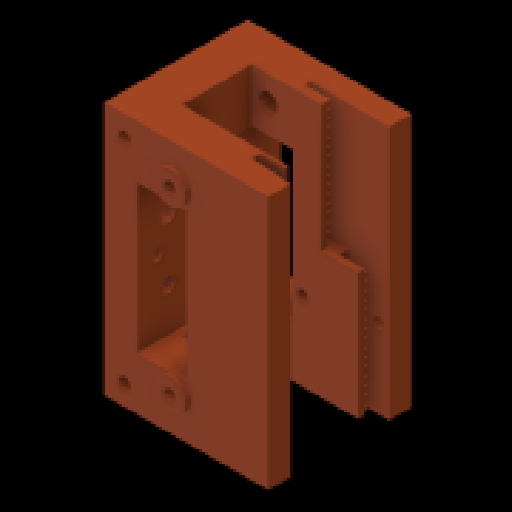
# Autodesk Inventor part: Toolhead Base
Saved by Autodesk Inventor 2023.3 (Build 273359000, 359)
## iProperties
Created: 2023-02-04
Part Number: Toolhead Base
Material: ABS Plastic
Document SubType Name: Modeling
Designer: remop
Density: 1.06 g/cm^3
Appearance: Smooth - Light Orange
Author: remop
Autodesk Inventor part; units mm, degrees
ref_plane "YZ Plane" through (0, 0, 0) normal (1, 0, 0) x (0, 1, 0)
ref_plane "XZ Plane" through (0, 0, 0) normal (0, 1, 0) x (-1, 0, 0)
ref_plane "XY Plane" through (0, 0, 0) normal (0, 0, 1) x (1, 0, 0)
sketch "Sketch1" plane through (0, 0, 0) normal (0, 0, 1) x (1, 0, 0)
  circle A0 centre (42.2396, 26.5) radius 2.25 projected
  circle A1 centre (42.2396, -23.5) radius 2.25 projected
  circle A2 centre (42.2396, -23.5) radius 6
  circle A3 centre (42.2396, 26.5) radius 6
  line L0 (48.2396, -23.5) -> (48.2396, -16.5)
  line L1 (48.2396, -16.5) -> (34.2396, -16.5)
  line L2 (34.2396, -16.5) -> (28.2396, -22.5)
  line L3 (28.2396, -22.5) -> (28.2396, -29.5)
  line L4 (28.2396, -29.5) -> (42.2396, -29.5)
  line L5 (48.2396, 26.5) -> (48.2396, 19.5)
  line L6 (48.2396, 19.5) -> (28.2396, 19.5)
  line L7 (28.2396, 19.5) -> (28.2396, 32.5)
  line L8 (28.2396, 32.5) -> (42.2396, 32.5)
  line L9 (42.2396, -29.5) -> (48.2396, -29.5)
  line L10 (48.2396, -29.5) -> (48.2396, -23.5)
  line L11 (48.2396, 26.5) -> (48.2396, 32.5)
  line L12 (48.2396, 32.5) -> (42.2396, 32.5)
  point P0 (0, 0)
  dimension "d0" = 12
  dimension "d3" = 14
  dimension "d4" = 45
  dimension "d5" = 7
  dimension "d6" = 7
  constraints: 26 end point, 8 tangent, 5 perpendicular, 5 point on circle, 3 horizontal, 2 centre point, 2 coincident, 2 point on line, 2 vertical, 1 collinear, 1 equal radius, 1 parallel, 1 vertical alignment
  measures "d0" diameter of A2
  measures "d3" distance of L3.end L4.end
  measures "d4" angle of L2 L3
  measures "d5" distance of L0.start L0.end
  measures "d6" distance of L2.end L3.end
extrude "Extrusion1" add sketch "Sketch1" along normal blind 9
sketch "Sketch2" plane through (0, 0, 9) normal (0, 0, 1) x (1, 0, 0)
  line L0 (28.2396, 32.5) -> (28.2396, 19.5) projected
  line L1 (28.2396, 19.5) -> (48.2396, 19.5) projected
  line L2 (48.2396, 19.5) -> (48.2396, 32.5) projected
  circle A0 centre (42.2396, 26.5) radius 2.25 projected
  line L3 (48.2396, -16.5) -> (34.2396, -16.5) projected
  line L4 (34.2396, -16.5) -> (28.2396, -22.5) projected
  line L5 (28.2396, -22.5) -> (28.2396, -29.5) projected
  line L6 (28.2396, -29.5) -> (48.2396, -29.5) projected
  circle A1 centre (42.2396, -23.5) radius 2.25 projected
  line L7 (36.2396, -15.705) -> (36.2396, 18.995) projected
  line L8 (36.2396, -15.705) -> (46.2396, -15.705) projected
  line L9 (46.2396, 18.995) -> (46.2396, -15.705) projected
  line L10 (36.2396, 18.995) -> (46.2396, 18.995) projected
  line L11 (34.2396, -16.5) -> (28.2396, -22.5) projected
  line L12 (28.2396, 19.5) -> (28.2396, -22.5)
  line L13 (36.2396, -15.705) -> (36.2396, -16.5)
  line L14 (36.2396, 18.995) -> (36.2396, 19.5)
  line L15 (28.2396, 19.5) -> (48.2396, 19.5) projected
  line L16 (38.2396, 19.5) -> (38.2396, 32.5)
  line L17 (48.2396, -16.5) -> (34.2396, -16.5) projected
  line L18 (38.2396, -16.5) -> (38.2396, -29.5)
  line L19 (28.2396, -29.5) -> (42.2396, -29.5) projected
  circle A2 centre (20.2396, -6.5) radius 14 projected
  circle A3 centre (20.2396, -6.5) radius 15
  line L20 (48.2396, -29.5) -> (48.2396, -16.5) projected
  line L21 (48.2396, 32.5) -> (28.2396, 32.5) projected
  point P0 (0, 0)
  point P1 (38.2396, 19.5)
  point P2 (35.2396, -6.5)
  point P3 (28.2396, -19.1886)
  point P4 (28.2396, 6.1886)
  dimension "d7" = 1
  constraints: 10 end point, 6 point on line, 2 midpoint, 1 centre point, 1 coincident, 1 collinear, 1 perpendicular, 1 vertical, 1 vertical alignment
  measures "d7" radial gap between concentric circles of A2 A3
extrude "Extrusion2" add sketch "Sketch2" along normal blind 10 contours L21 L16 L1 L0 | L1 L14 L7 L13 L3 L4 L12 A3 | L4 L3 L18 L6 L5
sketch "Sketch3" plane through (0, 0, 19) normal (0, 0, 1) x (1, 0, 0)
  line L0 (28.2396, -29.5) -> (38.2396, -29.5) projected
  line L1 (38.2396, -29.5) -> (38.2396, -16.5) projected
  line L2 (38.2396, -16.5) -> (36.2396, -16.5) projected
  line L3 (36.2396, -16.5) -> (36.2396, 19.5) projected
  line L4 (36.2396, 19.5) -> (38.2396, 19.5) projected
  line L5 (28.2396, 32.5) -> (28.2396, 6.1886) projected
  arc A0 (28.2396, -19.1886) -> (28.2396, 6.1886) centre (20.2396, -6.5) ccw projected
  line L6 (28.2396, -19.1886) -> (28.2396, -29.5) projected
  line L7 (28.2396, 19.5) -> (28.2396, 6.1886) projected
  line L8 (28.2396, -19.1886) -> (28.2396, -22.5) projected
  line L9 (28.2396, 6.1886) -> (28.2396, -19.1886)
  line L10 (38.2396, 32.5) -> (28.2396, 32.5) projected
  line L11 (38.2396, 19.5) -> (38.2396, 32.5) projected
  point P0 (0, 0)
  constraints: 2 end point, 1 vertical
extrude "Extrusion3" add sketch "Sketch3" along normal blind 12 contours L6 A0 L5 L10 L11 L4 L3 L2 L1 L0
sketch "Sketch5" plane through (0, 0, 9) normal (0, 0, -1) x (-1, 0, 0)
  line L0 (-28.2396, 19.5) -> (-36.2396, 19.5) projected
  line L1 (-36.2396, -16.5) -> (-36.2396, 19.5) projected
  line L2 (-36.2396, -16.5) -> (-34.2396, -16.5) projected
  line L3 (-34.2396, -16.5) -> (-28.2396, -22.5) projected
  line L4 (-28.2396, -19.1886) -> (-28.2396, -22.5) projected
  arc A0 (-28.2396, 6.1886) -> (-28.2396, -19.1886) centre (-20.2396, -6.5) ccw projected
  line L5 (-28.2396, 19.5) -> (-28.2396, 6.1886) projected
  arc A1 (-28.2396, 6.1886) -> (-28.2396, -19.1886) centre (-20.2396, -6.5) ccw projected
  line L6 (-31.2396, 3.698) -> (-36.2396, 3.698)
  line L7 (-36.2396, -16.5) -> (-36.2396, 19.5) projected
  point P0 (0, 0)
  dimension "d12" = 5
  constraints: 2 end point, 1 perpendicular, 1 point on circle, 1 point on line
  measures "d12" distance of L6.start L6.end
extrude "Extrusion4" add sketch "Sketch5" along normal up to surface (9 mm away) contours L5 A0 L6 L1 L0
sketch "Sketch7" plane through (0, 0, 31) normal (0, 0, 1) x (1, 0, 0)
  line L0 (28.2396, 32.5) -> (28.2396, 6.1886) projected
  arc A0 (28.2396, -19.1886) -> (28.2396, 6.1886) centre (20.2396, -6.5) ccw projected
  line L1 (28.2396, -19.1886) -> (28.2396, -29.5) projected
  line L2 (28.2396, -29.5) -> (38.2396, -29.5) projected
  line L3 (38.2396, -29.5) -> (38.2396, -16.5) projected
  line L4 (38.2396, -16.5) -> (36.2396, -16.5) projected
  line L5 (36.2396, -16.5) -> (36.2396, 19.5) projected
  line L6 (36.2396, 19.5) -> (38.2396, 19.5) projected
  line L7 (38.2396, 19.5) -> (38.2396, 32.5) projected
  line L8 (38.2396, 32.5) -> (28.2396, 32.5) projected
  arc A1 (31.2396, 3.698) -> (28.2396, 6.1886) centre (20.2396, -6.5) ccw projected
  line L9 (28.2396, -19.1886) -> (28.2396, 6.1886)
  point P0 (0, 0)
  constraints: 2 end point, 1 vertical
extrude "Extrusion5" add sketch "Sketch7" against normal blind 10 contours A0 L9
sketch "Sketch6" plane through (28.2396, 6.1886, 0) normal (-1, 0, 0) x (0, 0, 1)
  circle A0 centre (27.5, 2.9564) radius 1.2295 projected
  line L0 (0, 26.3114) -> (0, 0) projected
  line L1 (0, 0) -> (21, 0) projected
  line L2 (31, 26.3114) -> (31, -35.6886) projected
  line L3 (0, 26.3114) -> (31, 26.3114) projected
  circle A1 centre (7.5, 2.9564) radius 1.2295 projected
  circle A2 centre (27.5, -12.0436) radius 1.2295 projected
  circle A3 centre (7.5, -12.0436) radius 1.2295 projected
  line L4 (0, -28.6886) -> (0, -35.6886) projected
  line L5 (0, -35.6886) -> (31, -35.6886) projected
  line L6 (21, -25.3772) -> (21, 0) projected
  line L7 (9, -25.3772) -> (21, -25.3772) projected
  line L8 (9, -25.3772) -> (9, -28.6886) projected
  line L9 (0, -28.6886) -> (9, -28.6886) projected
  point P0 (0, -6.1886)
hole "Hole1" at (28.2396, -5.855, 27.5) at (28.2396, 9.145, 27.5) at (28.2396, 9.145, 7.5) direction (1, 0, 0) diameter 3.6 end through all counterbore diameter 6.5 counterbore depth 3.4 clearance for "Socket Head Cap Screw ISO 4762" size "M3" standard "ISO"
sketch "Sketch8" plane through (38.2396, -29.5, 9) normal (1, 0, 0) x (0, 0, -1)
  line L0 (0, 13) -> (0, 0) projected
  line L1 (0, 13) -> (-22, 13) projected
  line L2 (-22, 0) -> (-22, 13) projected
  line L3 (0, 0) -> (-22, 0) projected
  line L4 (0, 62) -> (0, 49) projected
  line L5 (0, 62) -> (-22, 62) projected
  line L6 (-22, 49) -> (-22, 62) projected
  line L7 (0, 49) -> (-22, 49) projected
  line L8 (-22, 49) -> (9, 49) projected
  line L9 (-26, 62) -> (-17, 62)
  line L10 (-17, 62) -> (-17, 49)
  line L11 (-17, 49) -> (-26, 49)
  line L12 (-26, 49) -> (-26, 62)
  line L13 (0, 13) -> (-22, 13) projected
  line L14 (-26, 0) -> (-17, 0)
  line L15 (-17, 0) -> (-17, 13)
  line L16 (-17, 13) -> (-26, 13)
  line L17 (-26, 13) -> (-26, 0)
  point P0 (9, 29.5)
  point P1 (-17, 49)
  point P2 (-17, 0)
  point P3 (-17, 13)
  dimension "d24" = 17
  dimension "d25" = 4
  constraints: 16 end point, 4 parallel, 3 point on line, 2 horizontal, 2 perpendicular, 1 vertical alignment
  measures "d24" distance between parallel lines of L15 L0
  measures "d25" distance between parallel lines of L17 L2
extrude "Extrusion6" add sketch "Sketch8" along normal up to surface (10 mm away) contours L15 L3 L2 L1 | L2 L14 L17 L16 | L10 L7 L6 L5 | L6 L11 L12 L9
sketch "Sketch9" plane through (0, 0, 31) normal (0, 0, 1) x (1, 0, 0)
  line L0 (28.2396, 32.5) -> (28.2396, -29.5) projected
  line L1 (28.2396, -29.5) -> (38.2396, -29.5) projected
  line L2 (38.2396, -29.5) -> (38.2396, -16.5) projected
  line L3 (38.2396, -16.5) -> (36.2396, -16.5) projected
  line L4 (36.2396, -16.5) -> (36.2396, 19.5) projected
  line L5 (36.2396, 19.5) -> (38.2396, 19.5) projected
  line L6 (38.2396, 19.5) -> (38.2396, 32.5) projected
  line L7 (38.2396, 32.5) -> (28.2396, 32.5) projected
  point P0 (0, 0)
extrude "Extrusion7" add sketch "Sketch9" along normal up to surface (4 mm away)
sketch "Sketch10" plane through (48.2396, 19.5, 26) normal (1, 0, 0) x (0, 0, -1)
  line L0 (0, 13) -> (0, 0) projected
  line L1 (-9, 13) -> (0, 13) projected
  line L2 (-9, 0) -> (-9, 13) projected
  line L3 (0, 0) -> (-9, 0) projected
  line L4 (-9, -49) -> (-9, -36) projected
  line L5 (0, -49) -> (-9, -49) projected
  line L6 (0, -36) -> (0, -49) projected
  line L7 (-9, -36) -> (0, -36) projected
  line L8 (26, -49) -> (26, -36) projected
  line L9 (26, -36) -> (17, -36) projected
  line L10 (17, -49) -> (17, -36) projected
  line L11 (26, -49) -> (17, -49) projected
  line L12 (26, 0) -> (26, 13) projected
  line L13 (26, 13) -> (17, 13) projected
  line L14 (17, 0) -> (17, 13) projected
  line L15 (26, 0) -> (17, 0) projected
  line L16 (26, 0) -> (26, -15.802) projected
  line L17 (26, 0) -> (26, -36)
  line L18 (17, -36) -> (17, -15.802) projected
  line L19 (17, -36) -> (17, 0)
  line L20 (0, 13) -> (0, 0) projected
  line L21 (0, 0) -> (0, -36)
  line L22 (17, -36) -> (-9, -36) projected
  line L23 (-9, -36) -> (-9, 0)
  point P0 (26, -19.5)
  constraints: 8 end point, 3 collinear, 1 perpendicular
extrude "Extrusion8" add sketch "Sketch10" along normal blind 1
sketch "Sketch11" plane through (49.2396, 19.5, 26) normal (1, 0, 0) x (0, 0, -1)
  line L0 (0, -49) -> (0, 13) projected
  line L1 (0, 13) -> (-9, 13) projected
  line L2 (-9, 13) -> (-9, -49) projected
  line L3 (-9, -49) -> (0, -49) projected
  line L4 (26, -49) -> (26, 13) projected
  line L5 (26, 13) -> (17, 13) projected
  line L6 (17, 13) -> (17, -49) projected
  line L7 (17, -49) -> (26, -49) projected
  line L8 (17, 13) -> (17, -49) projected
  line L9 (26, -36) -> (26, 0) projected
  line L10 (26, -18) -> (17, -18)
  line L11 (0, -49) -> (0, 13) projected
  line L12 (0, -18) -> (-9, -18)
  line L13 (-9, 0) -> (-9, -36) projected
  point P0 (0, -18)
  constraints: 4 end point, 4 midpoint
extrude "Extrusion9" add sketch "Sketch11" along normal blind 9 contours L12 L2 L1 L0 | L7 L6 L10 L4
sketch "Sketch12" plane through (49.2396, 19.5, 26) normal (1, 0, 0) x (0, 0, -1)
  line L0 (17, -18) -> (26, -18) projected
  line L1 (26, -18) -> (26, 13) projected
  line L2 (26, 13) -> (17, 13) projected
  line L3 (17, 13) -> (17, -18) projected
  line L4 (0, -18) -> (-9, -18) projected
  line L5 (-9, -18) -> (-9, -49) projected
  line L6 (-9, -49) -> (0, -49) projected
  line L7 (0, -49) -> (0, -18) projected
  line L8 (-3, -23) -> (-3, -163.2) projected
  line L9 (18.5, -13) -> (18.5, -18)
  line L10 (17, -18) -> (26, -18) projected
  line L11 (-3, -23) -> (-3, -18)
  line L12 (0, -18) -> (-9, -18) projected
  arc A0 (-2.5, -48) -> (-2.5, -47) centre (-2.5, -47.5) ccw
  arc A1 (-2.5, -48) -> (-2.5, -49) centre (-2.5, -48.5) ccw
  line L13 (-9, -49) -> (0, -49) projected
  line L14 (-2.5, -47) -> (-2.5, -49) construction
  line L15 (26, -49) -> (-9, -49) projected
  arc A2 (-2.5, -46) -> (-2.5, -45) centre (-2.5, -45.5) ccw
  arc A3 (-2.5, -46) -> (-2.5, -47) centre (-2.5, -46.5) ccw
  arc A4 (-2.5, -44) -> (-2.5, -43) centre (-2.5, -43.5) ccw
  arc A5 (-2.5, -44) -> (-2.5, -45) centre (-2.5, -44.5) ccw
  arc A6 (-2.5, -42) -> (-2.5, -41) centre (-2.5, -41.5) ccw
  arc A7 (-2.5, -42) -> (-2.5, -43) centre (-2.5, -42.5) ccw
  arc A8 (-2.5, -40) -> (-2.5, -39) centre (-2.5, -39.5) ccw
  arc A9 (-2.5, -40) -> (-2.5, -41) centre (-2.5, -40.5) ccw
  arc A10 (-2.5, -38) -> (-2.5, -37) centre (-2.5, -37.5) ccw
  arc A11 (-2.5, -38) -> (-2.5, -39) centre (-2.5, -38.5) ccw
  arc A12 (-2.5, -36) -> (-2.5, -35) centre (-2.5, -35.5) ccw
  arc A13 (-2.5, -36) -> (-2.5, -37) centre (-2.5, -36.5) ccw
  arc A14 (-2.5, -34) -> (-2.5, -33) centre (-2.5, -33.5) ccw
  arc A15 (-2.5, -34) -> (-2.5, -35) centre (-2.5, -34.5) ccw
  arc A16 (-2.5, -32) -> (-2.5, -31) centre (-2.5, -31.5) ccw
  arc A17 (-2.5, -32) -> (-2.5, -33) centre (-2.5, -32.5) ccw
  arc A18 (-2.5, -30) -> (-2.5, -29) centre (-2.5, -29.5) ccw
  arc A19 (-2.5, -30) -> (-2.5, -31) centre (-2.5, -30.5) ccw
  arc A20 (-2.5, -28) -> (-2.5, -27) centre (-2.5, -27.5) ccw
  arc A21 (-2.5, -28) -> (-2.5, -29) centre (-2.5, -28.5) ccw
  arc A22 (-2.5, -26) -> (-2.5, -25) centre (-2.5, -25.5) ccw
  arc A23 (-2.5, -26) -> (-2.5, -27) centre (-2.5, -26.5) ccw
  arc A24 (-2.5, -24) -> (-2.5, -23) centre (-2.5, -23.5) ccw
  arc A25 (-2.5, -24) -> (-2.5, -25) centre (-2.5, -24.5) ccw
  arc A26 (-2.5, -22) -> (-2.5, -21) centre (-2.5, -21.5) ccw
  arc A27 (-2.5, -22) -> (-2.5, -23) centre (-2.5, -22.5) ccw
  arc A28 (-2.5, -20) -> (-2.5, -19) centre (-2.5, -19.5) ccw
  arc A29 (-2.5, -20) -> (-2.5, -21) centre (-2.5, -20.5) ccw
  arc A30 (-2.5, -18) -> (-2.5, -17) centre (-2.5, -17.5) ccw
  arc A31 (-2.5, -18) -> (-2.5, -19) centre (-2.5, -18.5) ccw
  arc A32 (-2.5, -16) -> (-2.5, -15) centre (-2.5, -15.5) ccw
  arc A33 (-2.5, -16) -> (-2.5, -17) centre (-2.5, -16.5) ccw
  arc A34 (-2.5, -14) -> (-2.5, -13) centre (-2.5, -13.5) ccw
  arc A35 (-2.5, -14) -> (-2.5, -15) centre (-2.5, -14.5) ccw
  arc A36 (-2.5, -12) -> (-2.5, -11) centre (-2.5, -11.5) ccw
  arc A37 (-2.5, -12) -> (-2.5, -13) centre (-2.5, -12.5) ccw
  arc A38 (-2.5, -10) -> (-2.5, -9) centre (-2.5, -9.5) ccw
  arc A39 (-2.5, -10) -> (-2.5, -11) centre (-2.5, -10.5) ccw
  arc A40 (19, 12) -> (19, 13) centre (19, 12.5) ccw
  arc A41 (19, 12) -> (19, 11) centre (19, 11.5) ccw
  line L16 (26, 13) -> (-9, 13) projected
  line L17 (19, 13) -> (19, 11) construction
  line L18 (18.5, 127.2) -> (18.5, -13) projected
  arc A42 (19, 10) -> (19, 9) centre (19, 9.5) ccw
  arc A43 (19, 10) -> (19, 11) centre (19, 10.5) ccw
  arc A44 (19, 8) -> (19, 7) centre (19, 7.5) ccw
  arc A45 (19, 8) -> (19, 9) centre (19, 8.5) ccw
  arc A46 (19, 6) -> (19, 5) centre (19, 5.5) ccw
  arc A47 (19, 6) -> (19, 7) centre (19, 6.5) ccw
  arc A48 (19, 4) -> (19, 3) centre (19, 3.5) ccw
  arc A49 (19, 4) -> (19, 5) centre (19, 4.5) ccw
  arc A50 (19, 2) -> (19, 1) centre (19, 1.5) ccw
  arc A51 (19, 2) -> (19, 3) centre (19, 2.5) ccw
  arc A52 (19, 0) -> (19, -1) centre (19, -0.5) ccw
  arc A53 (19, 0) -> (19, 1) centre (19, 0.5) ccw
  arc A54 (19, -2) -> (19, -3) centre (19, -2.5) ccw
  arc A55 (19, -2) -> (19, -1) centre (19, -1.5) ccw
  arc A56 (19, -4) -> (19, -5) centre (19, -4.5) ccw
  arc A57 (19, -4) -> (19, -3) centre (19, -3.5) ccw
  arc A58 (19, -6) -> (19, -7) centre (19, -6.5) ccw
  arc A59 (19, -6) -> (19, -5) centre (19, -5.5) ccw
  arc A60 (19, -8) -> (19, -9) centre (19, -8.5) ccw
  arc A61 (19, -8) -> (19, -7) centre (19, -7.5) ccw
  arc A62 (19, -10) -> (19, -11) centre (19, -10.5) ccw
  arc A63 (19, -10) -> (19, -9) centre (19, -9.5) ccw
  arc A64 (19, -12) -> (19, -13) centre (19, -12.5) ccw
  arc A65 (19, -12) -> (19, -11) centre (19, -11.5) ccw
  arc A66 (19, -14) -> (19, -15) centre (19, -14.5) ccw
  arc A67 (19, -14) -> (19, -13) centre (19, -13.5) ccw
  arc A68 (19, -16) -> (19, -17) centre (19, -16.5) ccw
  arc A69 (19, -16) -> (19, -15) centre (19, -15.5) ccw
  arc A70 (19, -18) -> (19, -19) centre (19, -18.5) ccw
  arc A71 (19, -18) -> (19, -17) centre (19, -17.5) ccw
  line L19 (-1, -49) -> (-1, -18)
  line L20 (-9, -18) -> (0, -18) projected
  line L21 (26, 13) -> (17, 13) projected
  line L22 (20.5, -18) -> (20.5, 13)
  point P0 (26, -19.5)
  point P1 (19, 13)
  point P2 (-3, -49)
  point P3 (-2.5, -49)
  point P4 (-2.5, -18)
  point P5 (-2.5, -19)
  point P6 (-2.5, -21)
  point P7 (18.5, 13)
  point P8 (19, 11)
  point P9 (19, 9)
  point P10 (19, 7)
  point P11 (19, 5)
  point P12 (19, 3)
  point P13 (19, 1)
  point P14 (19, -1)
  point P15 (19, -3)
  point P16 (19, -5)
  point P17 (19, -7)
  point P18 (19, -9)
  point P19 (19, -11)
  point P20 (19, -13)
  point P21 (19, -15)
  point P22 (19, -17)
  point P23 (-3, -18.5)
  point P24 (-3, -20.5)
  point P25 (-3, -22.5)
  point P26 (-3, -24.5)
  point P27 (-3, -26.5)
  point P28 (-3, -28.5)
  point P29 (-3, -30.5)
  point P30 (-3, -32.5)
  point P31 (-3, -34.5)
  point P32 (-3, -36.5)
  point P33 (-3, -38.5)
  point P34 (-3, -40.5)
  point P35 (-3, -42.5)
  point P36 (-3, -44.5)
  point P37 (-3, -46.5)
  point P38 (-3, -48.5)
  point P39 (18.5, 11.5)
  point P40 (18.5, 9.5)
  point P41 (18.5, 7.5)
  point P42 (18.5, 5.5)
  point P43 (18.5, 3.5)
  point P44 (18.5, 1.5)
  point P45 (18.5, -0.5)
  point P46 (18.5, -2.5)
  point P47 (18.5, -4.5)
  point P48 (18.5, -6.5)
  point P49 (18.5, -8.5)
  point P50 (18.5, -10.5)
  point P51 (18.5, -12.5)
  point P52 (18.5, -14.5)
  point P53 (18.5, -16.5)
  point P54 (20.5, 13)
  dimension "d35" = 1
  dimension "d39" = 2
  dimension "d97" = 2
  dimension "d152" = 1.5
  dimension "d154" = 1.5
  constraints: 144 point on circle, 72 centre point, 12 end point, 8 point on line, 6 tangent, 4 perpendicular, 3 equal radius, 2 midpoint, 2 vertical, 2 vertical alignment, 1 coincident, 1 parallel, 238 other
  measures "d35" distance of A1.centre A0.centre
  measures "d39" distance of A0.centre A2.centre
  measures "d97" distance of A41.centre A42.centre
  measures "d152" distance from line of A28.centre L19
  measures "d154" distance from line of L22 A40.centre
extrude "Belts_Bottom" add sketch "Sketch12" along normal blind 6 contours L3 L2 L18 L9 L0 | L9 A66 A69 A68 | L2 A40 A41 L18 | L22 L2 L1 L0 | L9 L18 A64 A67 A66 | A41 A43 A42 L18 | A42 A45 A44 L18 | L18 A62 A65 A64 | A44 A47 A46 L18 | L18 A60 A63 A62 | A46 A49 A48 L18 | L18 A58 A61 A60 | A48 A51 A50 L18 | L18 A56 A59 A58 | A50 A53 A52 L18 | L18 A54 A57 A56 | A52 A55 A54 L18 | L7 L6 L19 L4 | L11 L8 L6 L5 L4 | A31 A28 A29 L11 | A29 A26 A27 L11 | L8 A3 A0 A1 | A27 A24 A25 L8 L11 | L8 A5 A2 A3 | L8 A7 A4 A5 | A25 A22 A23 L8 | L8 A9 A6 A7 | A23 A20 A21 L8 | L8 A11 A8 A9 | A21 A18 A19 L8 | L8 A13 A10 A11 | A19 A16 A17 L8 | L8 A15 A12 A13 | A17 A14 A15 L8
sketch "Sketch13" plane through (58.2396, 19.5, 26) normal (1, 0, 0) x (0, 0, -1)
  line L0 (-3, -13) -> (-3, 127.2) projected
  line L1 (-9, 13) -> (-9, -18) projected
  line L2 (-9, -18) -> (0, -18) projected
  line L3 (0, -18) -> (0, 13) projected
  line L4 (0, 13) -> (-9, 13) projected
  line L5 (26, -49) -> (26, -18) projected
  line L6 (26, -18) -> (17, -18) projected
  line L7 (17, -18) -> (17, -49) projected
  line L8 (17, -49) -> (26, -49) projected
  line L9 (-9, -18) -> (-3, -18) projected
  line L10 (-3, -13) -> (-3, -18)
  arc A0 (19, -48) -> (19, -49) centre (19, -48.5) ccw
  line L11 (17, -49) -> (26, -49) projected
  arc A1 (19, -48) -> (19, -47) centre (19, -47.5) ccw
  line L12 (19, -49) -> (19, -47) construction
  arc A2 (-2.5, 13) -> (-2.5, 12) centre (-2.5, 12.5) ccw
  line L13 (26, 13) -> (-9, 13) projected
  arc A3 (-2.5, 11) -> (-2.5, 12) centre (-2.5, 11.5) ccw
  line L14 (-2.5, 13) -> (-2.5, 11) construction
  arc A4 (-2.5, 9) -> (-2.5, 10) centre (-2.5, 9.5) ccw
  arc A5 (-2.5, 11) -> (-2.5, 10) centre (-2.5, 10.5) ccw
  arc A6 (-2.5, 7) -> (-2.5, 8) centre (-2.5, 7.5) ccw
  arc A7 (-2.5, 9) -> (-2.5, 8) centre (-2.5, 8.5) ccw
  arc A8 (-2.5, 5) -> (-2.5, 6) centre (-2.5, 5.5) ccw
  arc A9 (-2.5, 7) -> (-2.5, 6) centre (-2.5, 6.5) ccw
  arc A10 (-2.5, 3) -> (-2.5, 4) centre (-2.5, 3.5) ccw
  arc A11 (-2.5, 5) -> (-2.5, 4) centre (-2.5, 4.5) ccw
  arc A12 (-2.5, 1) -> (-2.5, 2) centre (-2.5, 1.5) ccw
  arc A13 (-2.5, 3) -> (-2.5, 2) centre (-2.5, 2.5) ccw
  arc A14 (-2.5, -1) -> (-2.5, 0) centre (-2.5, -0.5) ccw
  arc A15 (-2.5, 1) -> (-2.5, 0) centre (-2.5, 0.5) ccw
  arc A16 (-2.5, -3) -> (-2.5, -2) centre (-2.5, -2.5) ccw
  arc A17 (-2.5, -1) -> (-2.5, -2) centre (-2.5, -1.5) ccw
  arc A18 (-2.5, -5) -> (-2.5, -4) centre (-2.5, -4.5) ccw
  arc A19 (-2.5, -3) -> (-2.5, -4) centre (-2.5, -3.5) ccw
  arc A20 (-2.5, -7) -> (-2.5, -6) centre (-2.5, -6.5) ccw
  arc A21 (-2.5, -5) -> (-2.5, -6) centre (-2.5, -5.5) ccw
  arc A22 (-2.5, -9) -> (-2.5, -8) centre (-2.5, -8.5) ccw
  arc A23 (-2.5, -7) -> (-2.5, -8) centre (-2.5, -7.5) ccw
  arc A24 (-2.5, -11) -> (-2.5, -10) centre (-2.5, -10.5) ccw
  arc A25 (-2.5, -9) -> (-2.5, -10) centre (-2.5, -9.5) ccw
  arc A26 (-2.5, -13) -> (-2.5, -12) centre (-2.5, -12.5) ccw
  arc A27 (-2.5, -11) -> (-2.5, -12) centre (-2.5, -11.5) ccw
  arc A28 (-2.5, -15) -> (-2.5, -14) centre (-2.5, -14.5) ccw
  arc A29 (-2.5, -13) -> (-2.5, -14) centre (-2.5, -13.5) ccw
  arc A30 (-2.5, -17) -> (-2.5, -16) centre (-2.5, -16.5) ccw
  arc A31 (-2.5, -15) -> (-2.5, -16) centre (-2.5, -15.5) ccw
  arc A32 (-2.5, -19) -> (-2.5, -18) centre (-2.5, -18.5) ccw
  arc A33 (-2.5, -17) -> (-2.5, -18) centre (-2.5, -17.5) ccw
  line L15 (18.5, -163.2) -> (18.5, -23) projected
  line L16 (18.5, -23) -> (18.5, -18)
  arc A34 (19, -46) -> (19, -45) centre (19, -45.5) ccw
  arc A35 (19, -46) -> (19, -47) centre (19, -46.5) ccw
  arc A36 (19, -44) -> (19, -43) centre (19, -43.5) ccw
  arc A37 (19, -44) -> (19, -45) centre (19, -44.5) ccw
  arc A38 (19, -42) -> (19, -41) centre (19, -41.5) ccw
  arc A39 (19, -42) -> (19, -43) centre (19, -42.5) ccw
  arc A40 (19, -40) -> (19, -39) centre (19, -39.5) ccw
  arc A41 (19, -40) -> (19, -41) centre (19, -40.5) ccw
  arc A42 (19, -38) -> (19, -37) centre (19, -37.5) ccw
  arc A43 (19, -38) -> (19, -39) centre (19, -38.5) ccw
  arc A44 (19, -36) -> (19, -35) centre (19, -35.5) ccw
  arc A45 (19, -36) -> (19, -37) centre (19, -36.5) ccw
  arc A46 (19, -34) -> (19, -33) centre (19, -33.5) ccw
  arc A47 (19, -34) -> (19, -35) centre (19, -34.5) ccw
  arc A48 (19, -32) -> (19, -31) centre (19, -31.5) ccw
  arc A49 (19, -32) -> (19, -33) centre (19, -32.5) ccw
  arc A50 (19, -30) -> (19, -29) centre (19, -29.5) ccw
  arc A51 (19, -30) -> (19, -31) centre (19, -30.5) ccw
  arc A52 (19, -28) -> (19, -27) centre (19, -27.5) ccw
  arc A53 (19, -28) -> (19, -29) centre (19, -28.5) ccw
  arc A54 (19, -26) -> (19, -25) centre (19, -25.5) ccw
  arc A55 (19, -26) -> (19, -27) centre (19, -26.5) ccw
  arc A56 (19, -24) -> (19, -23) centre (19, -23.5) ccw
  arc A57 (19, -24) -> (19, -25) centre (19, -24.5) ccw
  arc A58 (19, -22) -> (19, -21) centre (19, -21.5) ccw
  arc A59 (19, -22) -> (19, -23) centre (19, -22.5) ccw
  arc A60 (19, -20) -> (19, -19) centre (19, -19.5) ccw
  arc A61 (19, -20) -> (19, -21) centre (19, -20.5) ccw
  arc A62 (19, -18) -> (19, -17) centre (19, -17.5) ccw
  arc A63 (19, -18) -> (19, -19) centre (19, -18.5) ccw
  line L17 (-1, 13) -> (-1, -18)
  line L18 (-9, -18) -> (0, -18) projected
  line L19 (20.5, 13) -> (20.5, -18) projected
  line L20 (20.5, -49) -> (20.5, -18)
  point P0 (26, -19.5)
  point P1 (-3, 13)
  point P2 (-2.5, 11)
  point P3 (-2.5, 9)
  point P4 (-2.5, 7)
  point P5 (-2.5, 5)
  point P6 (-2.5, 3)
  point P7 (-2.5, 1)
  point P8 (-2.5, -1)
  point P9 (-2.5, -3)
  point P10 (-2.5, -5)
  point P11 (-2.5, -7)
  point P12 (-2.5, -9)
  point P13 (-2.5, -11)
  point P14 (-2.5, -13)
  point P15 (-2.5, -15)
  point P16 (-2.5, -17)
  point P17 (-2.5, -18)
  point P18 (19, -18)
  point P19 (19, -19)
  point P20 (19, -21)
  point P21 (19, -23)
  point P22 (19, -25)
  point P23 (19, -27)
  point P24 (19, -29)
  point P25 (19, -31)
  point P26 (19, -33)
  point P27 (19, -35)
  point P28 (19, -37)
  point P29 (19, -39)
  point P30 (19, -41)
  point P31 (19, -43)
  point P32 (19, -45)
  point P33 (19, -47)
  point P34 (18.5, -49)
  point P35 (-3, 12.5)
  point P36 (-3, 10.5)
  point P37 (-3, 8.5)
  point P38 (-3, 6.5)
  point P39 (-3, 4.5)
  point P40 (-3, 2.5)
  point P41 (-3, 0.5)
  point P42 (-3, -1.5)
  point P43 (-3, -3.5)
  point P44 (-3, -5.5)
  point P45 (-3, -7.5)
  point P46 (-3, -9.5)
  point P47 (-3, -11.5)
  point P48 (-3, -13.5)
  point P49 (-3, -15.5)
  point P50 (-3, -17.5)
  point P51 (18.5, -18.5)
  point P52 (18.5, -20.5)
  point P53 (18.5, -22.5)
  point P54 (18.5, -24.5)
  point P55 (18.5, -26.5)
  point P56 (18.5, -28.5)
  point P57 (18.5, -30.5)
  point P58 (18.5, -32.5)
  point P59 (18.5, -34.5)
  point P60 (18.5, -36.5)
  point P61 (18.5, -38.5)
  point P62 (18.5, -40.5)
  point P63 (18.5, -42.5)
  point P64 (18.5, -44.5)
  point P65 (18.5, -46.5)
  point P66 (18.5, -48.5)
  dimension "d54" = 1
  dimension "d66" = 2
  dimension "d88" = 2
  dimension "d155" = 1.5
  dimension "d156" = 1.5
  constraints: 128 point on circle, 64 centre point, 12 end point, 6 point on line, 6 tangent, 5 vertical, 3 equal radius, 2 midpoint, 2 perpendicular, 2 vertical alignment, 210 other
  measures "d54" diameter of A0
  measures "d66" distance of A3.centre A4.centre
  measures "d88" distance of A1.centre A34.centre
  measures "d155" distance from line of L17 A24.centre
  measures "d156" distance from line of L20 A60.centre
extrude "Belts_Top" add sketch "Sketch13" along normal blind 6 contours L10 L2 L1 L4 L0 | L0 A27 A26 A29 L10 | L0 A25 A24 A27 | A29 A28 A31 L10 | L0 A23 A22 A25 | A31 A30 A33 L10 | L0 A21 A20 A23 | L0 A19 A18 A21 | L0 A17 A16 A19 | L17 L4 L3 L2 | L0 A15 A14 A17 | L0 A13 A12 A15 | L0 A11 A10 A13 | A2 A3 A5 L0 | L0 A9 A8 A11 | A5 A4 A7 L0 | L0 A7 A6 A9 | L8 L20 L6 L5 | L8 L7 L6 L16 L15 | L15 A35 A1 A0 | A63 A60 A61 L16 | L15 A37 A34 A35 | A61 A58 A59 L16 | L15 A39 A36 A37 | A59 A56 A57 L15 L16 | L15 A41 A38 A39 | L15 A43 A40 A41 | A57 A54 A55 L15 | L15 A45 A42 A43 | A55 A52 A53 L15 | L15 A47 A44 A45 | A53 A50 A51 L15 | L15 A49 A46 A47 | A51 A48 A49 L15
sketch "Sketch14" plane through (55.2396, 19.5, 26) normal (1, 0, 0) x (0, 0, -1)
  line L0 (-9, -49) -> (-3, -49) projected
  line L1 (-3, -18.5) -> (-3, -18) projected
  line L2 (-9, -18) -> (-3, -18) projected
  line L3 (-9, -18) -> (-9, -49) projected
  line L4 (26, 13) -> (20.5, 13) projected
  line L5 (26, -18) -> (20.5, -18) projected
  line L6 (26, -18) -> (26, 13) projected
  line L7 (19, 13) -> (17, 13) projected
  line L8 (17, 13) -> (17, -18) projected
  arc A0 (19, 12) -> (19, 13) centre (19, 12.5) ccw projected
  arc A1 (19, 10) -> (19, 11) centre (19, 10.5) ccw projected
  arc A2 (19, 8) -> (19, 9) centre (19, 8.5) ccw projected
  arc A3 (19, 6) -> (19, 7) centre (19, 6.5) ccw projected
  arc A4 (19, 4) -> (19, 5) centre (19, 4.5) ccw projected
  arc A5 (19, 2) -> (19, 3) centre (19, 2.5) ccw projected
  arc A6 (19, 0) -> (19, 1) centre (19, 0.5) ccw projected
  arc A7 (19, -2) -> (19, -1) centre (19, -1.5) ccw projected
  arc A8 (19, -4) -> (19, -3) centre (19, -3.5) ccw projected
  arc A9 (19, -6) -> (19, -5) centre (19, -5.5) ccw projected
  arc A10 (19, -8) -> (19, -7) centre (19, -7.5) ccw projected
  arc A11 (19, -10) -> (19, -9) centre (19, -9.5) ccw projected
  arc A12 (19, -12) -> (19, -11) centre (19, -11.5) ccw projected
  arc A13 (19, -14) -> (19, -13) centre (19, -13.5) ccw projected
  arc A14 (19, -16) -> (19, -15) centre (19, -15.5) ccw projected
  line L9 (18.5, -18) -> (17, -18) projected
  line L10 (26, -18) -> (19, -18) projected
  line L11 (21, -18) -> (21, 13)
  line L12 (26, 13) -> (-9, 13) projected
  line L13 (-3, -49) -> (-3, -48.5) projected
  arc A15 (-2.5, -48) -> (-3, -48.5) centre (-2.5, -48.5) ccw projected
  arc A16 (-2.5, -48) -> (-2.5, -47) centre (-2.5, -47.5) ccw projected
  arc A17 (-2.5, -46) -> (-2.5, -47) centre (-2.5, -46.5) ccw projected
  arc A18 (-2.5, -46) -> (-2.5, -45) centre (-2.5, -45.5) ccw projected
  arc A19 (-2.5, -44) -> (-2.5, -45) centre (-2.5, -44.5) ccw projected
  arc A20 (-2.5, -44) -> (-2.5, -43) centre (-2.5, -43.5) ccw projected
  arc A21 (-2.5, -42) -> (-2.5, -43) centre (-2.5, -42.5) ccw projected
  arc A22 (-2.5, -42) -> (-2.5, -41) centre (-2.5, -41.5) ccw projected
  arc A23 (-2.5, -40) -> (-2.5, -41) centre (-2.5, -40.5) ccw projected
  arc A24 (-2.5, -40) -> (-2.5, -39) centre (-2.5, -39.5) ccw projected
  arc A25 (-2.5, -38) -> (-2.5, -39) centre (-2.5, -38.5) ccw projected
  arc A26 (-2.5, -38) -> (-2.5, -37) centre (-2.5, -37.5) ccw projected
  arc A27 (-2.5, -36) -> (-2.5, -37) centre (-2.5, -36.5) ccw projected
  arc A28 (-2.5, -36) -> (-2.5, -35) centre (-2.5, -35.5) ccw projected
  arc A29 (-2.5, -34) -> (-2.5, -35) centre (-2.5, -34.5) ccw projected
  arc A30 (-2.5, -34) -> (-2.5, -33) centre (-2.5, -33.5) ccw projected
  arc A31 (-2.5, -32) -> (-2.5, -33) centre (-2.5, -32.5) ccw projected
  arc A32 (-2.5, -32) -> (-2.5, -31) centre (-2.5, -31.5) ccw projected
  arc A33 (-2.5, -30) -> (-2.5, -31) centre (-2.5, -30.5) ccw projected
  arc A34 (-2.5, -30) -> (-2.5, -29) centre (-2.5, -29.5) ccw projected
  arc A35 (-2.5, -28) -> (-2.5, -29) centre (-2.5, -28.5) ccw projected
  arc A36 (-2.5, -28) -> (-2.5, -27) centre (-2.5, -27.5) ccw projected
  arc A37 (-2.5, -26) -> (-2.5, -27) centre (-2.5, -26.5) ccw projected
  arc A38 (-2.5, -26) -> (-2.5, -25) centre (-2.5, -25.5) ccw projected
  arc A39 (-2.5, -24) -> (-2.5, -25) centre (-2.5, -24.5) ccw projected
  arc A40 (-2.5, -24) -> (-2.5, -23) centre (-2.5, -23.5) ccw projected
  arc A41 (-2.5, -22) -> (-2.5, -23) centre (-2.5, -22.5) ccw projected
  arc A42 (-2.5, -22) -> (-2.5, -21) centre (-2.5, -21.5) ccw projected
  arc A43 (-2.5, -20) -> (-2.5, -21) centre (-2.5, -20.5) ccw projected
  arc A44 (-2.5, -20) -> (-2.5, -19) centre (-2.5, -19.5) ccw projected
  arc A45 (-3, -18.5) -> (-2.5, -19) centre (-2.5, -18.5) ccw projected
  line L14 (18.5, -18) -> (18.5, -16.5) projected
  arc A46 (19, 12) -> (19, 11) centre (19, 11.5) ccw projected
  arc A47 (19, 10) -> (19, 9) centre (19, 9.5) ccw projected
  arc A48 (19, 8) -> (19, 7) centre (19, 7.5) ccw projected
  arc A49 (19, 6) -> (19, 5) centre (19, 5.5) ccw projected
  arc A50 (19, 4) -> (19, 3) centre (19, 3.5) ccw projected
  arc A51 (19, 2) -> (19, 1) centre (19, 1.5) ccw projected
  arc A52 (19, 0) -> (19, -1) centre (19, -0.5) ccw projected
  arc A53 (19, -2) -> (19, -3) centre (19, -2.5) ccw projected
  arc A54 (19, -4) -> (19, -5) centre (19, -4.5) ccw projected
  arc A55 (19, -6) -> (19, -7) centre (19, -6.5) ccw projected
  arc A56 (19, -8) -> (19, -9) centre (19, -8.5) ccw projected
  arc A57 (19, -10) -> (19, -11) centre (19, -10.5) ccw projected
  arc A58 (19, -12) -> (19, -13) centre (19, -12.5) ccw projected
  arc A59 (19, -14) -> (19, -15) centre (19, -14.5) ccw projected
  arc A60 (19, -16) -> (18.5, -16.5) centre (19, -16.5) ccw projected
  line L15 (20.5, 13) -> (20.5, -18) projected
  point P0 (26, -19.5)
  point P1 (18.5, 13)
  point P2 (21, 13)
  dimension "d102" = 5
  constraints: 2 end point, 2 point on line, 1 perpendicular
  measures "d102" distance between parallel lines of L6 L11
extrude "Walls" add sketch "Sketch14" along normal up to surface (9 mm away) contours L3 L2 L1 A45 A44 A43 A42 A41 A40 A39 A38 A37 A36 A35 A34 A33 A32 A31 A30 A29 A28 A27 A26 A25 A24 A23 A22 A21 A20 A19 A18 A17 A16 A15 L13 L0 | L6 L5 L11 L4 | L11 L5 L15 L4
sketch "Sketch18" plane through (28.2396, -29.5, 35) normal (0, 0, 1) x (1, 0, 0)
  line L0 (8, 13) -> (20, 13) projected
  line L1 (8, 49) -> (8, 13) projected
  line L2 (8, 49) -> (20, 49) projected
  line L3 (20, 49) -> (20, 13) projected
  line L4 (0, 0) -> (36, 0) projected
  line L5 (36, 62) -> (36, 0) projected
  line L6 (0, 62) -> (36, 62) projected
  line L7 (0, 0) -> (0, 62) projected
  circle A0 centre (17, 52.92) radius 1.75 projected
  circle A1 centre (17, 9.08) radius 1.75 projected
  circle A2 centre (17, 52.92) radius 3.92
  circle A3 centre (17, 9.08) radius 3.92
  circle A4 centre (17, 52.92) radius 1.4
  circle A5 centre (17, 9.08) radius 1.4
  point P0 (-28.2396, 29.5)
  dimension "d111" = 2.8
  constraints: 4 centre point, 4 coincident, 2 tangent, 1 equal radius
  measures "d111" diameter of A4
extrude "Extrusion15" add sketch "Sketch18" along normal blind 1 contours A2 | A3 | A0 | A1
sketch "Sketch19" plane through (28.2396, -29.5, 0) normal (-1, 0, 0) x (0, 0, 1)
  arc A0 (8.8498, 35.6886) -> (6.1502, 35.6886) centre (7.5, 38.645) ccw projected
  line L0 (8.8498, 35.6886) -> (21, 35.6886) projected
  line L1 (21, 10.3114) -> (21, 35.6886) projected
  line L2 (9, 10.3114) -> (21, 10.3114) projected
  line L3 (9, 10.3114) -> (9, 7) projected
  line L4 (0, 7) -> (9, 7) projected
  line L5 (0, 7) -> (0, 0) projected
  line L6 (0, 0) -> (35, 0) projected
  line L7 (35, 0) -> (35, 62) projected
  line L8 (0, 62) -> (35, 62) projected
  line L9 (0, 62) -> (0, 35.6886) projected
  line L10 (0, 35.6886) -> (6.1502, 35.6886) projected
  circle A1 centre (27.5, 23.645) radius 3.25 projected
  circle A2 centre (27.5, 38.645) radius 3.25 projected
  point P0 (0, 29.5)
  point P1 (5.0002, 52)
  point P2 (20, 52.0744)
  dimension "d112" = 15
  dimension "d113" = 20
  dimension "d114" = 10
  measures "d112" distance of point (20, 52.074) point (5, 52)
  measures "d113" distance from line of L9 point (20, 52.074)
  measures "d114" distance from line of point (5, 52) L8
hole "Hole2" at (28.2396, 22.5, 5.0002) at (28.2396, 22.5744, 20) direction (1, 0, 0) diameter 2.8 depth 9
sketch "Sketch20" plane through (28.2396, -29.5, 0) normal (-1, 0, 0) x (0, 0, 1)
  circle A0 centre (5.0002, 52) radius 1.4 projected
  circle A1 centre (20, 52.0744) radius 1.4 projected
  arc A2 (8.8498, 35.6886) -> (6.1502, 35.6886) centre (7.5, 38.645) ccw projected
  line L0 (8.8498, 35.6886) -> (21, 35.6886) projected
  line L1 (21, 10.3114) -> (21, 35.6886) projected
  line L2 (9, 10.3114) -> (21, 10.3114) projected
  line L3 (9, 10.3114) -> (9, 7) projected
  line L4 (0, 7) -> (9, 7) projected
  line L5 (0, 7) -> (0, 0) projected
  line L6 (0, 0) -> (35, 0) projected
  line L7 (35, 0) -> (35, 62) projected
  line L8 (0, 62) -> (35, 62) projected
  line L9 (0, 62) -> (0, 35.6886) projected
  line L10 (0, 35.6886) -> (6.1502, 35.6886) projected
  circle A3 centre (27.5, 23.645) radius 3.25 projected
  circle A4 centre (27.5, 38.645) radius 3.25 projected
  point P0 (0, 29.5)
  point P1 (30, 11.145)
  point P2 (30, 31.145)
  dimension "d122" = 15
  dimension "d123" = 7.5
  dimension "d124" = 5
  dimension "d125" = 20
  constraints: 1 vertical alignment
  measures "d122" distance of A4.centre A3.centre
  measures "d123" vertical distance of A3.centre point (30, 31.145)
  measures "d124" distance from line of L7 point (30, 31.145)
  measures "d125" distance of point (30, 11.145) point (30, 31.145)
hole "Hole3" at (28.2396, -18.355, 30) at (28.2396, 1.645, 30) direction (1, 0, 0) diameter 2.8 depth 8 tip angle 118
sketch "Sketch24" plane through (64.2396, 19.5, 26) normal (1, 0, 0) x (0, 0, -1)
  line L0 (-3, -17.5) -> (-3, -18.5) projected
  arc A0 (-2.5, -17) -> (-3, -17.5) centre (-2.5, -17.5) ccw projected
  arc A1 (-2.5, -17) -> (-2.5, -16) centre (-2.5, -16.5) ccw projected
  arc A2 (-2.5, -15) -> (-2.5, -16) centre (-2.5, -15.5) ccw projected
  arc A3 (-2.5, -15) -> (-2.5, -14) centre (-2.5, -14.5) ccw projected
  arc A4 (-2.5, -13) -> (-2.5, -14) centre (-2.5, -13.5) ccw projected
  arc A5 (-2.5, -13) -> (-2.5, -12) centre (-2.5, -12.5) ccw projected
  arc A6 (-2.5, -11) -> (-2.5, -12) centre (-2.5, -11.5) ccw projected
  arc A7 (-2.5, -11) -> (-2.5, -10) centre (-2.5, -10.5) ccw projected
  arc A8 (-2.5, -9) -> (-2.5, -10) centre (-2.5, -9.5) ccw projected
  arc A9 (-2.5, -9) -> (-2.5, -8) centre (-2.5, -8.5) ccw projected
  arc A10 (-2.5, -7) -> (-2.5, -8) centre (-2.5, -7.5) ccw projected
  arc A11 (-2.5, -7) -> (-2.5, -6) centre (-2.5, -6.5) ccw projected
  arc A12 (-2.5, -5) -> (-2.5, -6) centre (-2.5, -5.5) ccw projected
  arc A13 (-2.5, -5) -> (-2.5, -4) centre (-2.5, -4.5) ccw projected
  arc A14 (-2.5, -3) -> (-2.5, -4) centre (-2.5, -3.5) ccw projected
  arc A15 (-2.5, -3) -> (-2.5, -2) centre (-2.5, -2.5) ccw projected
  arc A16 (-2.5, -1) -> (-2.5, -2) centre (-2.5, -1.5) ccw projected
  arc A17 (-2.5, -1) -> (-2.5, 0) centre (-2.5, -0.5) ccw projected
  arc A18 (-2.5, 1) -> (-2.5, 0) centre (-2.5, 0.5) ccw projected
  arc A19 (-2.5, 1) -> (-2.5, 2) centre (-2.5, 1.5) ccw projected
  arc A20 (-2.5, 3) -> (-2.5, 2) centre (-2.5, 2.5) ccw projected
  arc A21 (-2.5, 3) -> (-2.5, 4) centre (-2.5, 3.5) ccw projected
  arc A22 (-2.5, 5) -> (-2.5, 4) centre (-2.5, 4.5) ccw projected
  arc A23 (-2.5, 5) -> (-2.5, 6) centre (-2.5, 5.5) ccw projected
  arc A24 (-2.5, 7) -> (-2.5, 6) centre (-2.5, 6.5) ccw projected
  arc A25 (-2.5, 7) -> (-2.5, 8) centre (-2.5, 7.5) ccw projected
  arc A26 (-2.5, 9) -> (-2.5, 8) centre (-2.5, 8.5) ccw projected
  arc A27 (-2.5, 9) -> (-2.5, 10) centre (-2.5, 9.5) ccw projected
  arc A28 (-2.5, 11) -> (-2.5, 10) centre (-2.5, 10.5) ccw projected
  arc A29 (-2.5, 11) -> (-2.5, 12) centre (-2.5, 11.5) ccw projected
  arc A30 (-3, 12.5) -> (-2.5, 12) centre (-2.5, 12.5) ccw projected
  line L1 (-3, 12.5) -> (-3, 13) projected
  line L2 (-3, 13) -> (-9, 13) projected
  line L3 (-9, 13) -> (-9, -49) projected
  line L4 (-3, -49) -> (-9, -49) projected
  line L5 (-3, -48.5) -> (-3, -49) projected
  arc A31 (-2.5, -48) -> (-3, -48.5) centre (-2.5, -48.5) ccw projected
  arc A32 (-2.5, -48) -> (-2.5, -47) centre (-2.5, -47.5) ccw projected
  arc A33 (-2.5, -46) -> (-2.5, -47) centre (-2.5, -46.5) ccw projected
  arc A34 (-2.5, -46) -> (-2.5, -45) centre (-2.5, -45.5) ccw projected
  arc A35 (-2.5, -44) -> (-2.5, -45) centre (-2.5, -44.5) ccw projected
  arc A36 (-2.5, -44) -> (-2.5, -43) centre (-2.5, -43.5) ccw projected
  arc A37 (-2.5, -42) -> (-2.5, -43) centre (-2.5, -42.5) ccw projected
  arc A38 (-2.5, -42) -> (-2.5, -41) centre (-2.5, -41.5) ccw projected
  arc A39 (-2.5, -40) -> (-2.5, -41) centre (-2.5, -40.5) ccw projected
  arc A40 (-2.5, -40) -> (-2.5, -39) centre (-2.5, -39.5) ccw projected
  arc A41 (-2.5, -38) -> (-2.5, -39) centre (-2.5, -38.5) ccw projected
  arc A42 (-2.5, -38) -> (-2.5, -37) centre (-2.5, -37.5) ccw projected
  arc A43 (-2.5, -36) -> (-2.5, -37) centre (-2.5, -36.5) ccw projected
  arc A44 (-2.5, -36) -> (-2.5, -35) centre (-2.5, -35.5) ccw projected
  arc A45 (-2.5, -34) -> (-2.5, -35) centre (-2.5, -34.5) ccw projected
  arc A46 (-2.5, -34) -> (-2.5, -33) centre (-2.5, -33.5) ccw projected
  arc A47 (-2.5, -32) -> (-2.5, -33) centre (-2.5, -32.5) ccw projected
  arc A48 (-2.5, -32) -> (-2.5, -31) centre (-2.5, -31.5) ccw projected
  arc A49 (-2.5, -30) -> (-2.5, -31) centre (-2.5, -30.5) ccw projected
  arc A50 (-2.5, -30) -> (-2.5, -29) centre (-2.5, -29.5) ccw projected
  arc A51 (-2.5, -28) -> (-2.5, -29) centre (-2.5, -28.5) ccw projected
  arc A52 (-2.5, -28) -> (-2.5, -27) centre (-2.5, -27.5) ccw projected
  arc A53 (-2.5, -26) -> (-2.5, -27) centre (-2.5, -26.5) ccw projected
  arc A54 (-2.5, -26) -> (-2.5, -25) centre (-2.5, -25.5) ccw projected
  arc A55 (-2.5, -24) -> (-2.5, -25) centre (-2.5, -24.5) ccw projected
  arc A56 (-2.5, -24) -> (-2.5, -23) centre (-2.5, -23.5) ccw projected
  arc A57 (-2.5, -22) -> (-2.5, -23) centre (-2.5, -22.5) ccw projected
  arc A58 (-2.5, -22) -> (-2.5, -21) centre (-2.5, -21.5) ccw projected
  arc A59 (-2.5, -20) -> (-2.5, -21) centre (-2.5, -20.5) ccw projected
  arc A60 (-2.5, -20) -> (-2.5, -19) centre (-2.5, -19.5) ccw projected
  arc A61 (-3, -18.5) -> (-2.5, -19) centre (-2.5, -18.5) ccw projected
  line L6 (20.5, -49) -> (20.5, 13) projected
  line L7 (20.5, -49) -> (26, -49) projected
  line L8 (26, -49) -> (26, 13) projected
  line L9 (20.5, 13) -> (26, 13) projected
  line L10 (-3, 13) -> (-9, 13) projected
  line L11 (-3.5, 13) -> (-3.5, -49)
  point P0 (26, -19.5)
  point P1 (-3.5, 13)
  dimension "d157" = 5.5
  dimension "d158" = 5.5
  constraints: 2 end point, 2 point on line, 1 perpendicular
  measures "d157" distance between parallel lines of L8 L6
  measures "d158" distance between parallel lines of L3 L11
extrude "Extrusion17" add sketch "Sketch24" along normal blind 4 contours L11 L4 L3 L2 | L6 L9 L8 L7
sketch "Sketch22" plane through (0, 0, 0) normal (0, 0, -1) x (-1, 0, 0)
  circle A0 centre (-65.7396, -10.2) radius 1.5 projected
  circle A1 centre (-50.7396, -10.2) radius 1.5 projected
  point P0 (0, 0)
hole "Hole4" at (65.7396, -10.2, 0) at (50.7396, -10.2, 0) direction (0, 0, 1) diameter 2.7 depth 10 tip angle 118
sketch "Sketch23" plane through (28.2396, -29.5, 35) normal (0, 0, 1) x (1, 0, 0)
  line L0 (0, 62) -> (36, 62) projected
  circle A0 centre (17, 9.08) radius 1.75 projected
  circle A1 centre (17, 52.92) radius 1.75 projected
  line L1 (0, 0) -> (0, 62) projected
  line L2 (8.25, 0) -> (40, 0) projected
  line L3 (0, 0) -> (40, 0) projected
  point P0 (-28.2396, 29.5)
  point P1 (5, 57)
  point P2 (5, 5)
  dimension "d142" = 5
  dimension "d144" = 5
  dimension "d163" = 5
  constraints: 1 vertical alignment
  measures "d142" distance from line of L1 point (5, 5)
  measures "d144" distance from line of L0 point (5, 57)
  measures "d163" distance from line of L3 point (5, 5)
hole "Hole5" at (33.2396, 27.5, 35) at (33.2396, -24.5, 35) at (45.2396, 23.42, 35) at (45.2396, -20.42, 35) direction (0, 0, -1) diameter 2.8 depth 9 tip angle 118
sketch "Sketch25" plane through (31.6396, 9.145, 27.5) normal (-1, 0, 0) x (0, 0, 1)
  circle A0 centre (0, -15) radius 1.8 projected
  circle A1 centre (0, 0) radius 1.8 projected
  circle A2 centre (-20, 0) radius 1.8 projected
  point P0 (-27.5, -9.145)
extrude "Extrusion18" add sketch "Sketch25" against normal blind 0.2
equation "\"d144\" = d143"
equation "\"d143\" = 5"
body "Solid1"
